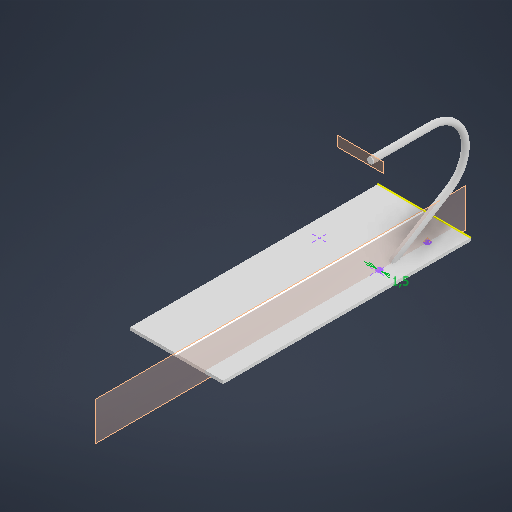
# Autodesk Inventor part: my_portafilter_holder_2
Saved by Autodesk Inventor 2026 (Build 300175000, 175)
## iProperties
Created: 2025-04-15
Part Number: my_portafilter_holder_2
Material: Generic
Document SubType Name: Modeling
Designer: Paul Juschitz
Density: 1 g/cm^3
Appearance: Default
Author: Paul Juschitz
Autodesk Inventor part; units mm, degrees
ref_plane "XZ Plane" through (0, 0, 0) normal (0, 1, 0) x (-1, 0, 0)
sketch "Sketch1" plane through (0, 0, 0) normal (0, 1, 0) x (-1, 0, 0)
  line L0 (0, 0) -> (30, 0)
  line L1 (30, 0) -> (30, 80)
  line L2 (30, 80) -> (0, 80)
  line L3 (0, 80) -> (0, 0)
  dimension "d0" = 30
  dimension "d1" = 80
  constraints: 8 end point, 2 parallel, 1 horizontal, 1 perpendicular
  measures "d0" distance of L2.end L1.end
  measures "d1" distance of L1.end L0.end
extrude "Extrusion1" add sketch "Sketch1" along normal blind 1
sketch "Sketch2" plane through (0, 1, 0) normal (0, 1, 0) x (1, 0, 0)
  line L0 (0, 0) -> (-30, 0) projected
  line L1 (-15, 0) -> (-15, -80.2026)
  circle A0 centre (-5.7061, -23.8105) radius 0.75
  circle A1 centre (-5.7061, -8.252) radius 0.7509
  point P0 (-5.7061, -24.5605)
  point P1 (-24.2939, -24.5605)
  dimension "d8" = 1.5
  constraints: 2 end point, 1 centre point, 1 midpoint, 1 symmetric about line, 1 vertical, 1 vertical alignment, 2 other
ref_plane "Work Plane1" through (-5.7061, 1, 24.5605) normal (1, 0, 0) x (0, 1, 0)
sketch "Sketch3" plane through (-5.7061, 1, 24.5605) normal (1, 0, 0) x (0, 1, 0)
  line L0 (0, -24.5605) -> (0, 55.4395)
  line L1 (3.6849, -4.2162) -> (14.4816, -21.8449)
  line L2 (27.4947, -17.9201) -> (27.4947, 1.6769)
  arc A0 (14.4816, -21.8449) -> (27.4947, -17.9201) centre (20.3963, -17.9201) ccw
  arc A1 (3.6849, -4.2162) -> (-0.8754, -1.0746) centre (-1.7465, -7.2198) ccw
  point P0 (-1, -24.5605)
  constraints: 6 end point, 4 point on circle, 2 centre point, 1 tangent
ref_plane "Work Plane2" through (0, 0, 26) normal (0, 0, 1) x (1, 0, 0)
sketch "Sketch5" plane through (0, 0, 26) normal (0, 0, 1) x (1, 0, 0)
  circle A0 centre (-6.2222, 32.5528) radius 1
  point P0 (0, 0)
  dimension "d20" = 2
  constraints: 1 centre point
  measures "d20" diameter of A0
sweep "Sweep5" add profiles "Sketch5" path "Sketch3" separate body path curves L2 A0 L1 A1
equation "\"d2\" = thickness"
equation "\"thickness\" = 1"
body "Solid1"
body "Solid3"
